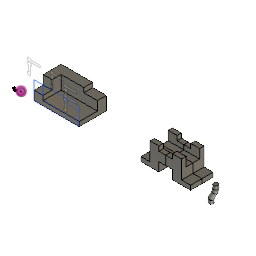
a97a6294-5307-49d0-b536-01d9514b3983 (Autodesk Fusion 360 design; units mm, degrees)
Autodesk Fusion 360 part; units mm, degrees
note: some values were not read from the file. Chosen so that the rebuilt part matches the saved one: which bodies a step acts on; which face or edge a step refers to. Set by a fixed rule: which sketch regions a step uses.
sketch "Sketch1" plane through (0, 0, 0) normal (0, 1, 0) x (1, 0, 0)
sketch "Sketch2" plane through (0, 0, 0) normal (0, 1, 0) x (1, 0, 0)
  line L0 (0, 0) -> (-4, 0)
  line L1 (-4, 0) -> (-4, -2.25)
  line L2 (-4, -2.25) -> (-2.5, -2.25)
  line L3 (-2.5, -2.25) -> (-2.5, -1.5)
  line L4 (-2.5, -1.5) -> (-1.25, -1.5)
  line L5 (-1.25, -1.5) -> (-1.25, -0.75)
  line L6 (-1.25, -0.75) -> (0, -0.75)
  line L7 (0, -0.75) -> (0, 0)
  dimension "d3" = 4
  dimension "d4" = 2.25
  dimension "d5" = 1.5
  dimension "d6" = 1.25
  dimension "d7" = 0.75
  dimension "d8" = 0.75
  dimension "d9" = 0.75
  measures "d3" distance of L0.start
extrude "Extrude1" add sketch "Sketch2" along normal blind 1.25 makes body 1
sketch "Sketch3" plane through (0, 0, 0) normal (0, 1, 0) x (1, 0, 0)
  line L0 (14.6457, 1.203) -> (114.6457, 1.203)
  line L1 (114.6457, 1.203) -> (114.6457, -38.797)
  line L2 (114.6457, -38.797) -> (14.6457, -38.797)
  line L3 (14.6457, -38.797) -> (14.6457, 1.203)
  line L4 (84.6457, -38.797) -> (84.6457, -28.797)
  line L5 (84.6457, -28.797) -> (114.6457, -28.797)
  line L6 (34.6457, -38.797) -> (34.6457, -8.797)
  line L7 (34.6457, -8.797) -> (114.6457, -8.797)
  line L8 (14.6457, -38.797) -> (34.6457, -38.797)
  line L9 (34.6457, -38.797) -> (34.6457, -18.797)
  line L10 (34.6457, -18.797) -> (14.6457, -18.797)
  line L11 (14.6457, -18.797) -> (14.6457, -38.797)
  dimension "d12" = 40
  dimension "d13" = 100
  dimension "d16" = 30
  dimension "d17" = 10
  dimension "d23" = 10
  dimension "d24" = 20
  dimension "d25" = 100
  dimension "d26" = 20
  measures "d13" distance of origin
  measures "d23" distance of L0 L7
  measures "d24" distance of L3 L6
  measures "d25" distance of origin
extrude "Extrude3" add sketch "Sketch3" along normal blind 60 separate body contours L0 L1 L3 L6 L7 L10 | L2 L3 L6 L8 L9 L10 L11 | L1 L2 L4 L5 L6 L7 L9 makes body 2
extrude "Extrude2" add sketch "Sketch3" along normal blind 60 separate body contours L0 L1 L3 L6 L7 L10 | L2 L3 L6 L8 L9 L10 L11 | L1 L2 L4 L5 L6 L7 L9 makes body 3
extrude "Extrude4" cut sketch "Sketch3" along normal blind 20 contours L2 L3 L6 L8 L9 L10 L11 bodies 2 3
extrude "Extrude5" cut sketch "Sketch3" along normal blind 40 contours L1 L2 L4 L5 L6 L7 L9 bodies 2 3
sketch "Sketch4" plane through (0, 0, 0) normal (0, 1, 0) x (1, 0, 0)
  line L0 (250, 0) -> (250, -10)
  line L1 (250, -10) -> (270, -10)
  line L2 (270, -10) -> (270, -50)
  line L3 (270, -50) -> (290, -50)
  line L4 (290, -50) -> (290, -40)
  line L5 (290, -40) -> (305, -40)
  line L6 (305, -40) -> (305, -20)
  line L7 (305, -20) -> (290, -20)
  line L8 (290, -20) -> (290, 0)
  line L9 (290, 0) -> (250, 0)
  dimension "d42" = 15
  dimension "d43" = 20
  dimension "d44" = 15
  dimension "d45" = 20
  dimension "d46" = 40
  dimension "d47" = 10
  dimension "d48" = 40
  dimension "d54" = 10
  measures "d42" distance of origin
  measures "d43" distance of origin
  measures "d46" distance of origin
  measures "d47" distance of origin
extrude "Extrude6" add sketch "Sketch4" along normal blind 25 separate body makes body 4
sketch "Sketch5" plane through (0, 25, 0) normal (0, 1, 0) x (-1, 0, 0)
  line L0 (-290, 0) -> (-250, 0)
  line L1 (-250, 0) -> (-250, 10)
  line L2 (-250, 10) -> (-270, 10)
  line L3 (-270, 10) -> (-270, 50)
  line L4 (-270, 50) -> (-290, 50)
  line L5 (-290, 50) -> (-290, 40)
  line L6 (-290, 40) -> (-305, 40)
  line L7 (-305, 40) -> (-305, 20)
  line L8 (-305, 20) -> (-290, 20)
  line L9 (-290, 20) -> (-290, 0)
  line L10 (-305, 29.9973) -> (-270, 30)
  dimension "d52" = 0.004
  dimension "d53" = 20
  measures "d52" angle of L4 L10
extrude "Extrude7" cut sketch "Sketch5" against normal blind 15 contours L3 L4 L5 L6 L7 L10 bodies 4
mirror "Mirror1" about plane through (0, 25, 0) normal (0, 1, 0) of bodies 4 makes body 5
mirror "Mirror2" about plane through (305, 0, 40) normal (1, 0, 0) of bodies 4 5 makes body 6 at (333.3333, 50, 26.6667) makes body 7 at (333.3333, 0, 26.6667)
sketch "Sketch6" plane through (0, 0, 0) normal (0, -1, 0) x (1, 0, 0)
  line L0 (320, 0) -> (360, 0)
  line L1 (360, 0) -> (360, 10)
  line L2 (360, 10) -> (340, 10)
  line L3 (340, 10) -> (340, 50)
  line L4 (340, 50) -> (320, 50)
  line L5 (320, 50) -> (320, 40)
  line L6 (320, 40) -> (305, 40)
  line L7 (305, 40) -> (305, 20)
  line L8 (305, 20) -> (320, 20)
  line L9 (320, 20) -> (320, 0)
  line L10 (410, 40) -> (410, 32.3607)
  line L11 (400, 7.6393) -> (400, 0)
  line L12 (408.9443, 27.8885) -> (401.0557, 12.1115)
  arc A0 (401.0557, 12.1115) -> (400, 7.6393) centre (410, 7.6393) ccw
  arc A1 (408.9443, 27.8885) -> (410, 32.3607) centre (400, 32.3607) ccw
  dimension "d59" = 10
  dimension "d60" = 10
  dimension "d61" = 10
  measures "d60" radius of A0
  measures "d61" radius of A1
sketch "Sketch7" plane through (0, 0, 0) normal (0, 0, 1) x (1, 0, 0)
  circle A0 centre (405.5, 0) radius 5.5
sweep "Sweep1" add profiles "Sketch7" path "Sketch6" along L10 A1 L12 A0 L11 section 1 separate body makes body 8
sketch "Sketch8" plane through (0, 0, 0) normal (0, 1, 0) x (1, 0, 0)
sketch "Sketch9" plane through (0, 0, 0) normal (0, 0, 1) x (1, 0, 0)
  line L0 (-17.5, 1.5) -> (-17.5, 1.5)
  line L1 (-16.5, 0.5) -> (-13, 0.5)
  line L2 (-13, 0.5) -> (-13, 1.5)
  line L3 (-4, 0) -> (-2.5, 0)
  line L4 (-17.5, 1.5) -> (-13, 1.5)
  arc A0 (-17, 1.5) -> (-16, 1.5) centre (-16.5, 1.5) ccw
  arc A1 (-17.5, 1.5) -> (-16.5, 0.5) centre (-16.5, 1.5) ccw
  dimension "d68" = 1
  dimension "d69" = 4.5
  dimension "d70" = 0.5
  dimension "d71" = 1
  measures "d70" distance of L1 L3
  measures "d71" radius of A1
extrude "Extrude8" add sketch "Sketch9" along normal blind 0.5 separate body contours L1 L2 L4 A0 A1 makes body 9
sketch "Sketch10" plane through (0, 0, 0.5) normal (0, 0, 1) x (-1, 0, 0)
  line L0 (17, -1.5) -> (17.5, -1.5)
  arc A0 (17.5, -1.5) -> (16.5, -0.5) centre (16.5, -1.5) ccw
  line L1 (16.5, -0.5) -> (13, -0.5)
  line L2 (13, -0.5) -> (13, -1.5)
  line L3 (13, -1.5) -> (16, -1.5)
  arc A1 (17, -1.5) -> (16, -1.5) centre (16.5, -1.5) ccw
  line L4 (13, -0.5) -> (15, -0.5)
  line L5 (15, -0.5) -> (15, -1)
  line L6 (15, -1) -> (13, -1)
  line L7 (13, -1) -> (13, -0.5)
  dimension "d74" = 2
extrude "Extrude9" add sketch "Sketch10" along normal blind 2 contours L1 L2 L4 L5 L6 L7 bodies 9
sketch "Sketch11" plane through (0, 0.5, 0) normal (0, -1, 0) x (1, 0, 0)
  line L0 (-16.5, 0) -> (-13, 0)
  line L1 (-13, 0) -> (-13, 2.5)
  line L2 (-13, 2.5) -> (-15, 2.5)
  line L3 (-15, 2.5) -> (-15, 0.5)
  line L4 (-15, 0.5) -> (-16.5, 0.5)
  line L5 (-16.5, 0.5) -> (-16.5, 0)
sketch "Sketch12" plane through (-14.75, 0.5, 1.25) normal (0, -1, 0) x (1, 0, 0)
  line L0 (1.75, 1.25) -> (-0.25, 1.25)
  point P0 (0, -20)
fillet "Fillet1" radius 1 1 edges at (-15, 0.75, 2.5) on bodies 9
fillet "Fillet2" radius 1 1 edges at (-13, 0.75, 2.5) on bodies 9
hole "Hole1" at (-14, 0.5, 1.5) direction (0, 1, 0) diameter 1 depth 0.7 tip angle 118 bodies 9
mirror "Mirror3" about plane through (-16, 1.5, 0) normal (0, 1, 0) of bodies 9 makes body 10
sketch "Sketch13" plane through (0, 0.5, 0) normal (0, -1, 0) x (1, 0, 0)
  circle A0 centre (-27.5, 0) radius 4
  circle A1 centre (-27.5, 0) radius 1.1
  circle A2 centre (-27.5, 2.5) radius 0.7
  circle A3 centre (-29.2678, 1.7678) radius 0.7
  circle A4 centre (-30, 0) radius 0.7
  circle A5 centre (-29.2678, -1.7678) radius 0.7
  circle A6 centre (-27.5, -2.5) radius 0.7
  circle A7 centre (-25.7322, -1.7678) radius 0.7
  circle A8 centre (-25, 0) radius 0.7
  circle A9 centre (-25.7322, 1.7678) radius 0.7
  dimension "d83" = 8
  dimension "d84" = 2.2
  dimension "d85" = 1.4
  dimension "d87" = 360
  measures "d83" diameter of A0
  measures "d84" diameter of A1
  measures "d85" diameter of A2
extrude "Extrude10" add sketch "Sketch13" along normal blind 2 separate body makes body 11
